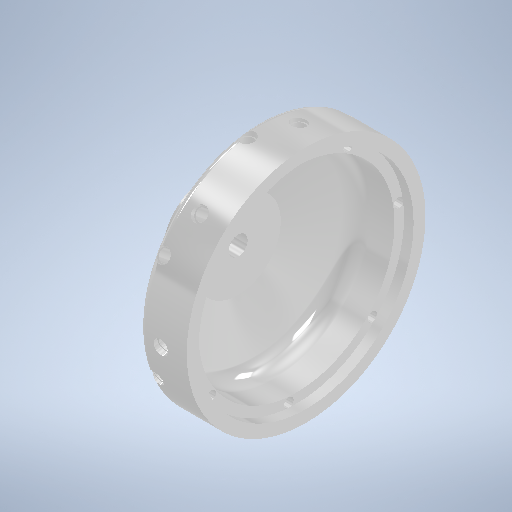
# Autodesk Inventor part: sonnenrad
Saved by Autodesk Inventor 2025 (Build 290162010, 162A)
## iProperties
Created: 2024-07-16
Part Number: sonnenrad
Material: Aluminum 6061-AHC
Document SubType Name: Modeling
Designer: ffogue
Density: 2.7 g/cm^3
Appearance: Aluminium - dunkel
Author: ffogue
Autodesk Inventor part; units mm, degrees
ref_plane "YZ Plane" through (0, 0, 0) normal (1, 0, 0) x (0, 1, 0)
sketch "Skizze1" plane through (0, 0, 0) normal (0, 1, 0) x (-1, 0, 0)
  line L0 (0, 0) -> (0, 18)
  line L1 (0, 18) -> (-7, 18)
  arc A0 (-9.9896, 18.5796) -> (-7, 18) centre (-7, 26) ccw
  line L2 (-9.9896, 18.5796) -> (-22.233, 48.1477)
  line L3 (-25.0048, 50) -> (-42, 50)
  line L4 (-42, 50) -> (-42, 0)
  line L5 (-42, 0) -> (0, 0)
  arc A1 (-22.233, 48.1477) -> (-25.0048, 50) centre (-25.0048, 47) ccw
  line L6 (-22.233, 48.1477) -> (-25.732, 56.5978) construction
  line L7 (-25.0048, 50) -> (-19.2372, 50) construction
  point P0 (-23.3379, 49.4943)
  point P1 (-23, 50)
  dimension "d1" = 42
  dimension "d2" = 8
  dimension "d3" = 3
  dimension "d4" = 100
  dimension "d5" = 36
  dimension "d7" = 19
  dimension "d8" = 35
  constraints: 16 end point, 5 point on circle, 3 perpendicular, 3 tangent, 2 centre point, 2 point on line, 1 collinear, 1 horizontal, 1 parallel, 1 vertical
  measures "d1" distance between parallel lines of L4 L0
  measures "d2" radius of A0
  measures "d3" radius of A1
  measures "d4" diameter of L3 L5
  measures "d5" diameter of L1 L5
  measures "d7" distance from line of L4 point (-23, 50)
  measures "d8" distance from line of L4 A0.centre
revolve "Umdrehung1" add sketch "Skizze1" angle 360 about axis through (42, 0, 0) along (-1, 0, 0)
sketch "Skizze2" plane through (0, 0, 0) normal (0, 1, 0) x (-1, 0, 0)
  line L0 (-42, 50) -> (-25.0048, 50) projected
  line L1 (-22.233, 48.1477) -> (-9.9896, 18.5796) projected
  line L2 (-22.233, -48.1477) -> (-9.9896, -18.5796) projected
  arc A0 (-25.0048, -50) -> (-22.233, -48.1477) centre (-25.0048, -47) ccw projected
  line L3 (-42, -50) -> (-25.0048, -50) projected
  arc A1 (-22.233, 48.1477) -> (-25.0048, 50) centre (-25.0048, 47) ccw projected
  line L4 (-42, -50) -> (-42, 50) projected
  line L5 (-13.4896, 0) -> (-13.4896, 17.8836)
  line L6 (-13.4896, 17.8836) -> (-21.0162, 36.0606)
  arc A2 (-21.0162, 36.0606) -> (-28.4076, 41) centre (-28.4076, 33) ccw
  line L7 (-28.4076, 41) -> (-38, 41)
  line L8 (-25.0048, -50) -> (-25.0048, 50) projected
  line L9 (-38, 41) -> (-38, 45)
  line L10 (-38, 45) -> (-42, 45)
  line L11 (-13.4896, 0) -> (-42, 0)
  point P0 (0, 0)
  dimension "d11" = 4
  dimension "d12" = 8
  dimension "d13" = 3.5
  dimension "d14" = 82
  dimension "d15" = 90
  dimension "d16" = 3.5
  constraints: 12 end point, 3 perpendicular, 2 point on circle, 2 tangent, 1 centre point, 1 horizontal alignment, 1 midpoint, 1 parallel, 1 point on line, 1 vertical
  measures "d11" distance of L9.end L10.end
  measures "d12" radius of A2
  measures "d13" distance between parallel lines of L6 L1
  measures "d14" diameter of L7 L11
  measures "d15" diameter of L10 L11
  measures "d16" horizontal distance of L5.end L1.end
revolve "Umdrehung2" cut sketch "Skizze2" angle 360 about axis through (13.4896, 0, 0) along (1, 0, 0) contours L10 L9 L7 A2 L8 L11 L4 | A2 L6 L5 L11 L8
sketch "Skizze3" plane through (0, 0, 0) normal (-1, 0, 0) x (0, 0, 1)
  circle A0 centre (0, 0) radius 18 projected
  point P0 (0, 0)
  constraints: 1 coincident
hole "Bohrung1" at (0, 0, 0) direction (1, 0, 0) diameter 8 depth 13.4896 counterbore diameter 28 counterbore depth 8
ref_plane "Arbeitsebene1" through (0, 0, 50) normal (0, 0, 1) x (1, 0, 0)
ref_plane "Arbeitsebene2" through (19.1, 0, 0) normal (-1, 0, 0) x (0, -1, 0)
sketch "Skizze5" plane through (19.1, 0, 0) normal (-1, 0, 0) x (0, -1, 0)
  circle A0 centre (0, 0) radius 45 projected
  circle A1 centre (0, 0) radius 50 projected
  circle A2 centre (0, 0) radius 43.25 construction
  line L0 (0, 0) -> (0, 60.825) construction
  line L1 (0, 0) -> (-21.625, 37.4556) construction
  point P0 (0, 0)
  dimension "d36" = 86.5
  dimension "d37" = 30
  constraints: 4 end point, 2 coincident, 1 vertical, 3 other
  measures "d37" angle of L0 L1
hole "Bohrung2" at (19.1, 21.625, 37.4556) direction (1, 0, 0) diameter 4 depth 18.9 counterbore diameter 7 counterbore depth 2.3
pattern_circular "Runde Anordnung1" count 7 over 360 about axis through (40, 0, 0) along (-1, 0, 0) of "Bohrung2"
sketch "Skizze7" plane through (0, 0, 50) normal (0, 0, 1) x (1, 0, 0)
  line L0 (0, 0) -> (42.0441, 0) construction
  line L1 (42, 50) -> (42, -50) projected
  point P0 (25.5, -8)
  dimension "d41" = 16.5
  dimension "d42" = 8
  constraints: 2 end point, 1 horizontal
  measures "d41" distance from line of L1 point (25.5, -8)
  measures "d42" distance from line of L0 point (25.5, -8)
hole "Bohrung3" at (25.5, -8, 50) direction (0, 0, -1) diameter 5 depth 9 counterbore diameter 6 counterbore depth 2.3
pattern_circular "Runde Anordnung2" count 7 over 360 about axis through (40, 0, 0) along (-1, 0, 0) of "Bohrung3"
sketch "Skizze8" plane through (0, 0, 50) normal (0, 0, 1) x (1, 0, 0)
  line L0 (0, 0) -> (41.8727, 0) construction
  circle A0 centre (25.5, -8) radius 2.5 projected
  line L1 (42, 50) -> (42, -50) projected
  point P0 (31, 8)
  dimension "d53" = 16
  dimension "d54" = 11
  constraints: 2 end point, 1 horizontal
  measures "d53" vertical distance of point (31, 8) A0.centre
  measures "d54" distance from line of L1 point (31, 8)
hole "Bohrung4" at (31, 8, 50) direction (0, 0, -1) diameter 5 depth 9 counterbore diameter 6 counterbore depth 2.3
pattern_circular "Runde Anordnung3" count 7 over 360 about axis through (40, 0, 0) along (-1, 0, 0) of "Bohrung4"
equation "\"d16\" = d13"
